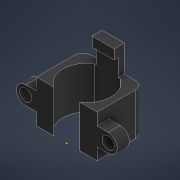
# Autodesk Inventor part: Suporte Externo - Motor
Saved by Autodesk Inventor 2021 (Build 250183000, 183)
## iProperties
Created: 2021-02-03
Part Number: Suporte Externo - Motor
Material: Genérico
Document SubType Name: Modeling
Designer: João
Density: 1 g/cm^3
Appearance: Borracha - Preta
Author: João
Autodesk Inventor part; units mm, degrees
ref_plane "YZ Plane" through (0, 0, 0) normal (1, 0, 0) x (0, 1, 0)
sketch "Esboço1" plane through (0, 0, 0) normal (0, 1, 0) x (-1, 0, 0)
  line L0 (-7.5, 0) -> (-7.5, -11.5)
  line L1 (-7.5, -11.5) -> (7.5, -11.5)
  line L2 (7.5, -11.5) -> (7.5, 0)
  line L3 (-6, -10) -> (-6, 0)
  line L4 (6, 0) -> (6, -10)
  line L5 (6, -10) -> (-6, -10)
  line L6 (7.5, 0) -> (6, 0)
  line L7 (-6, 0) -> (-7.5, 0)
  arc A0 (-3.2499, 0) -> (-3.2501, -10) centre (-0.0795, -5.0001) ccw
  line L8 (-3.2501, -10) -> (3.2501, -10)
  arc A1 (3.2501, -10) -> (3.2499, 0) centre (0.0795, -5.0001) ccw
  line L9 (3.2499, 0) -> (-3.2499, 0)
  line L10 (6, -10) -> (-6, -10)
  line L11 (-6, -10) -> (-6, 0)
  line L12 (-6, 0) -> (6, 0)
  line L13 (6, 0) -> (6, -10)
  point P0 (0, 0)
  point P1 (-3.2499, 0)
  dimension "d0" = 15
  dimension "d1" = 11.5
  dimension "d2" = 1.5
  dimension "d3" = 11.5
  constraints: 28 end point, 4 point on circle, 3 horizontal, 3 parallel, 2 centre point, 2 vertical, 1 perpendicular
  measures "d0" distance of L2.start L0.end
  measures "d1" distance of L0.end L7.end
  measures "d2" distance between parallel lines of L1 L5
  measures "d3" distance between parallel lines of L1 L6
extrude "Extrusão1" add sketch "Esboço1" along normal blind 13.5 contours L7 L3 L5 L4 L6 L2 L1 L0 | L12 A0 L3 | A0 L5 L3 | L12 L4 A1 | A1 L4 L5
sketch "Esboço2" plane through (0, 13.5, 0) normal (0, 1, 0) x (1, 0, 0)
  line L0 (-3.2501, 10) -> (3.2501, 10) projected
  line L1 (7.5, 11.5) -> (-7.5, 11.5) projected
  line L2 (-3.2501, 10) -> (3.2499, 10)
  line L3 (3.2499, 10) -> (3.2499, 11.5)
  line L4 (3.2499, 11.5) -> (-3.2501, 11.5)
  line L5 (-3.2501, 11.5) -> (-3.2501, 10)
  point P0 (0, 0)
  dimension "d8" = 6.5
  constraints: 8 end point, 2 parallel, 1 horizontal, 1 perpendicular, 1 point on line
  measures "d8" distance of L4.end L3.end
extrude "Extrusão2" add sketch "Esboço2" along normal blind 5
sketch "Esboço3" plane through (-3.2501, 0, -10) normal (0, 0, 1) x (1, 0, 0)
  line L0 (0, 13.5) -> (0, 18.5) projected
  line L1 (6.5, 13.5) -> (6.5, 18.5) projected
  line L2 (0, 14.8) -> (6.5, 14.8)
  line L3 (6.5, 14.8) -> (6.5, 15.3)
  line L4 (6.5, 15.3) -> (0, 15.3)
  line L5 (0, 15.3) -> (0, 14.8)
  line L6 (6.5, 18.5) -> (0, 18.5) projected
  line L7 (0, 18.5) -> (6.5, 18.5)
  line L8 (6.5, 18.5) -> (6.5, 18)
  line L9 (6.5, 18) -> (0, 18)
  line L10 (0, 18) -> (0, 18.5)
  line L11 (0, 17.2) -> (6.5, 17.2)
  line L12 (6.5, 17.2) -> (6.5, 16.7)
  line L13 (6.5, 16.7) -> (0, 16.7)
  line L14 (0, 16.7) -> (0, 17.2)
  point P0 (3.2501, 0)
  point P1 (0, 15.3)
  point P2 (6.5, 14.8)
  point P3 (0, 16.7)
  point P4 (6.5, 17.2)
  dimension "d11" = 0.5
  dimension "d12" = 0.5
  dimension "d13" = 0.5
  constraints: 24 end point, 6 parallel, 5 point on line, 3 horizontal, 3 perpendicular
  measures "d11" distance of L3.end L2.end
  measures "d12" distance of L7.end L8.end
  measures "d13" distance of L11.end L12.end
extrude "Extrusão3" add sketch "Esboço3" along normal blind 1 contours L0 L4 L1 L2 | L0 L6 L1 L9
extrude "Extrusão4" add sketch "Esboço3" along normal blind 0.5 contours L0 L11 L1 L13
sketch "Esboço4" plane through (0, 13.5, 0) normal (0, 1, 0) x (1, 0, 0)
  line L0 (-3.2501, 10) -> (-3.2501, 11.5) projected
  line L1 (-3.2501, 11.5) -> (-7.5, 11.5) projected
  line L2 (-7.5, 11.5) -> (-7.5, 0) projected
  line L3 (-7.5, 0) -> (-3.2499, 0) projected
  arc A0 (-3.2501, 10) -> (-3.2499, 0) centre (-0.0795, 5.0001) ccw projected
  line L4 (3.2499, 11.5) -> (3.2499, 10) projected
  line L5 (3.2499, 10) -> (3.2501, 10) projected
  arc A1 (3.2499, 0) -> (3.2501, 10) centre (0.0795, 5.0001) ccw projected
  line L6 (3.2499, 0) -> (7.5, 0) projected
  line L7 (7.5, 0) -> (7.5, 11.5) projected
  line L8 (7.5, 11.5) -> (3.2499, 11.5) projected
  line L9 (-3.2501, 9) -> (3.2499, 9) projected
  line L10 (-3.2501, 11.5) -> (-2.7501, 11.5)
  line L11 (-2.7501, 11.5) -> (-2.7501, 9)
  line L12 (-2.7501, 9) -> (-3.2501, 9)
  line L13 (-3.2501, 9) -> (-3.2501, 11.5)
  line L14 (3.2499, 11.5) -> (2.7499, 11.5)
  line L15 (2.7499, 11.5) -> (2.7499, 9)
  line L16 (2.7499, 9) -> (3.2499, 9)
  line L17 (3.2499, 9) -> (3.2499, 11.5)
  point P0 (0, 0)
  dimension "d20" = 0.5
  dimension "d21" = 0.5
  constraints: 16 end point, 4 parallel, 2 horizontal, 2 perpendicular, 2 point on line
  measures "d20" distance of L11.end L12.end
  measures "d21" distance of L16.end L15.end
extrude "Extrusão5" cut sketch "Esboço4" against normal blind 3 contours A0 L3 L2 L1 L0 | L8 L7 L6 A1 L4
sketch "Esboço5" plane through (0, 18.5, 0) normal (0, 1, 0) x (1, 0, 0)
  line L0 (-7.5, 11.5) -> (-3.2501, 11.5) projected
  line L1 (-3.2501, 9) -> (3.2499, 9) projected
  line L2 (-3.2501, 11.5) -> (-2.7501, 11.5)
  line L3 (-2.7501, 11.5) -> (-2.7501, 9)
  line L4 (-2.7501, 9) -> (-3.2501, 9)
  line L5 (-3.2501, 9) -> (-3.2501, 11.5)
  line L6 (3.2499, 11.5) -> (3.2499, 9) projected
  line L7 (3.2499, 11.5) -> (2.7499, 11.5)
  line L8 (2.7499, 11.5) -> (2.7499, 9)
  line L9 (2.7499, 9) -> (3.2499, 9)
  line L10 (3.2499, 9) -> (3.2499, 11.5)
  point P0 (0, 0)
  dimension "d22" = 0.5
  dimension "d23" = 0.5
  constraints: 16 end point, 4 parallel, 2 horizontal, 2 perpendicular, 2 point on line
  measures "d22" distance of L3.end L4.end
  measures "d23" distance of L9.end L8.end
extrude "Extrusão6" cut sketch "Esboço5" against normal up to surface (8 mm away)
sketch "Esboço6" plane through (3.2499, 0, 0) normal (0, 0, 1) x (1, 0, 0)
  point P0 (-3.2499, 0)
ref_plane "Plano de trabalho1" through (3.2499, 0, 0) normal (0, 0, 1) x (1, 0, 0)
sketch "Esboço7" plane through (3.2499, 0, 0) normal (0, 0, 1) x (1, 0, 0)
  line L0 (4.2501, 0) -> (4.2501, 10.5) projected
  line L1 (4.2501, 10.5) -> (4.2501, 0)
  circle A0 centre (6.9929, 5.2499) radius 1.5
  circle A1 centre (6.9929, 5.2499) radius 2.25
  line L2 (6.9929, 7.4999) -> (4.2501, 7.4999)
  line L3 (6.9929, 2.9999) -> (4.2501, 2.9999)
  line L4 (4.2501, 5.2499) -> (4.7429, 5.2499)
  line L5 (5.4929, 5.2499) -> (9.7501, 5.2499)
  point P0 (-3.2499, 0)
  dimension "d28" = 3
  dimension "d29" = 4.5
  constraints: 10 end point, 4 point on line, 3 horizontal, 3 point on circle, 1 centre point, 1 coincident, 1 collinear, 1 horizontal alignment, 1 perpendicular, 1 tangent, 2 other
  measures "d29" diameter of A1
extrude "Extrusão7" add sketch "Esboço7" against normal blind 3
ref_plane "Plano de trabalho2" through (-7.5, 0, 0) normal (0, 0, 1) x (1, 0, 0)
sketch "Esboço8" plane through (-7.5, 0, 0) normal (0, 0, 1) x (1, 0, 0)
  circle A0 centre (17.7428, 5.2499) radius 1.5
  line L0 (15, 10.5) -> (10.7499, 10.5) projected
  line L1 (10.7499, 0) -> (10.7499, 10.5) projected
  line L2 (10.7499, 0) -> (15, 0) projected
  line L3 (15, 0) -> (15, 2.9999) projected
  line L4 (15, 2.9999) -> (17.7428, 2.9999) projected
  arc A1 (17.7428, 2.9999) -> (17.7428, 7.4999) centre (17.7428, 5.2499) ccw projected
  line L5 (17.7428, 7.4999) -> (15, 7.4999) projected
  line L6 (15, 7.4999) -> (15, 10.5) projected
  circle A2 centre (-2.7428, 5.2499) radius 1.5
  line L7 (0, 0) -> (0, 2.9999)
  line L8 (0, 2.9999) -> (-2.7428, 2.9999)
  arc A3 (-2.7428, 7.4999) -> (-2.7428, 2.9999) centre (-2.7428, 5.2499) ccw
  line L9 (-2.7428, 7.4999) -> (0, 7.4999)
  line L10 (0, 7.4999) -> (0, 10.5)
  line L11 (0, 0) -> (0, 10.5) projected
  line L12 (0, 10.5) -> (0, 0)
  point P0 (7.5, 0)
  constraints: 10 end point, 3 centre point, 2 point on circle, 1 vertical
extrude "Extrusão8" add sketch "Esboço8" against normal blind 3 contours L8 A3 L9 L11
sketch "Esboço9" plane through (7.5, 0, -11.5) normal (0, 0, -1) x (-1, 0, 0)
  line L0 (10.2501, 18) -> (10.2501, 17.2) projected
  line L1 (10.2501, 17.2) -> (4.7501, 17.2) projected
  line L2 (4.7501, 17.2) -> (4.7501, 18) projected
  line L3 (4.7501, 18) -> (10.2501, 18) projected
  line L4 (10.2501, 18.5) -> (10.2501, 18) projected
  line L5 (10.2501, 18) -> (4.7501, 18) projected
  line L6 (4.7501, 18) -> (4.7501, 18.5) projected
  line L7 (4.7501, 18.5) -> (10.2501, 18.5) projected
  point P0 (7.5, 0)
extrude "Extrusão9" cut sketch "Esboço9" against normal blind 10
sketch "Esboço10" plane through (-2.7501, 15.3, -10) normal (0, 0, 1) x (1, 0, 0)
  line L0 (0, 1.4) -> (0, 0) projected
  line L1 (0, 0) -> (5.5, 0) projected
  line L2 (5.5, 0) -> (5.5, 1.4) projected
  line L3 (5.5, 1.4) -> (0, 1.4) projected
  line L4 (0, 1.9) -> (0, 1.4) projected
  line L5 (0, 1.4) -> (5.5, 1.4) projected
  line L6 (5.5, 1.4) -> (5.5, 1.9) projected
  line L7 (5.5, 1.9) -> (0, 1.9) projected
  point P0 (2.7501, -15.3)
extrude "Extrusão10" add sketch "Esboço10" along normal up to surface (1 mm away)
fillet "Arredondamento1" radius 2 2 edges at (7.5, 5.25, -11.5) (-7.5, 5.25, -11.5)
